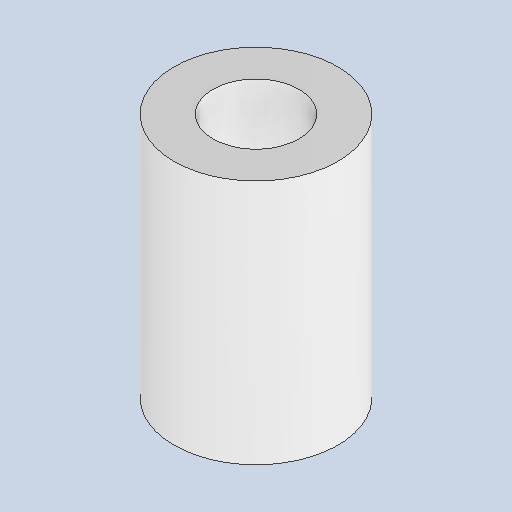
# Autodesk Inventor part: C-2006-4
Saved by Autodesk Inventor 2024.2 (Build 282272000, 272)
## iProperties
Created: 2024-01-28
Part Number: C-2006-4
Material: Acetal Resin, White
Document SubType Name: Modeling
Designer: Masato Kubotera
Density: 1.425 g/cm^3
Appearance: Smooth - White
Vendor: HIROSUGI
Catalog Web Link: https://www.hirosugi-net.co.jp/shop/g/g5920/
Author: Masato Kubotera
Autodesk Inventor part; units mm, degrees
ref_plane "YZ Plane" through (0, 0, 0) normal (1, 0, 0) x (0, 1, 0)
ref_plane "XZ Plane" through (0, 0, 0) normal (0, 1, 0) x (-1, 0, 0)
ref_plane "XY Plane" through (0, 0, 0) normal (0, 0, 1) x (1, 0, 0)
sketch "Sketch1" plane through (0, 0, 0) normal (0, 1, 0) x (-1, 0, 0)
  line L0 (0, 0) -> (0, 6) construction
  line L1 (-1.05, 0) -> (-2, 0)
  line L2 (-2, 0) -> (-2, 6)
  line L3 (-2, 6) -> (-1.05, 6)
  line L4 (-1.05, 6) -> (-1.05, 0)
  dimension "d0" = 6
  dimension "d1" = 2.1
  dimension "d2" = 4
  constraints: 10 end point, 2 parallel, 2 point on line, 1 horizontal, 1 perpendicular, 1 vertical
  measures "d0" distance of L0.start L0.end
  measures "d1" diameter of L4 L0
  measures "d2" diameter of L2 L0
revolve "Revolution1" add sketch "Sketch1" angle 360 about axis through (0, 0, 0) along (0, 0, 1)
body "Solid1"
